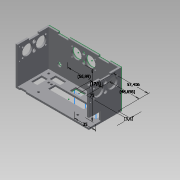
# Autodesk Inventor part: Kepala
Saved by Autodesk Inventor 2015 SP1 (Build 190203100, 203)
## iProperties
Created: 2015-02-01
Part Number: Kepala
Material: Generic
Document SubType Name: Modeling
Designer: Rafi Kurnia Putra
Density: 1 g/cm^3
Appearance: Default
Mass: 66.641 g
Surface Area: 406.742 cm^2
Volume: 66.641 cm^3
Author: Rafi Kurnia Putra
Autodesk Inventor part; units mm, degrees
ref_plane "YZ Plane" through (0, 0, 0) normal (1, 0, 0) x (0, 1, 0)
ref_plane "XY Plane" through (0, 0, 0) normal (0, 0, 1) x (1, 0, 0)
sketch "Sketch1" plane through (0, 0, 0) normal (0, 1, 0) x (-1, 0, 0)
  line L0 (60.406, -27.1071) -> (-60.406, -27.1071)
  line L1 (-60.406, -27.1071) -> (-60.406, 27.1071)
  line L2 (-60.406, 27.1071) -> (60.406, 27.1071)
  line L3 (60.406, 27.1071) -> (60.406, -27.1071)
  line L4 (60.406, -27.1071) -> (-60.406, 27.1071) construction
  line L5 (-60.406, -27.1071) -> (60.406, 27.1071) construction
  line L6 (-57.406, 24.1071) -> (-57.406, -27.1071)
  line L7 (57.406, -27.1071) -> (57.406, 24.1071)
  line L8 (57.406, 24.1071) -> (-57.406, 24.1071)
  point P0 (0, 0)
  point P1 (0, 0)
  dimension "d49" = 120.812
  dimension "d51" = 3
  dimension "d57" = 3
  dimension "d58" = 3
  dimension "d59" = 114.812
  dimension "d61" = 51.2141
  constraints: 18 end point, 3 midpoint, 3 parallel, 2 point on line, 1 horizontal, 1 perpendicular, 1 other
  measures "d49" distance of L1.end L2.end
  measures "d51" distance between parallel lines of L6 L1
  measures "d57" distance between parallel lines of L7 L3
  measures "d58" distance between parallel lines of L8 L2
  measures "d59" distance between parallel lines of L7 L6
  measures "d61" distance between parallel lines of L8 L0
extrude "Extrusion5" add sketch "Sketch1" against normal blind 3
extrude "Extrusion6" add sketch "Sketch1" along normal blind 60 contours L0 L7 L8 L6 L1 L2 L3
sketch "Sketch6" plane through (0, -3, 0) normal (0, -1, 0) x (1, 0, 0)
  circle A0 centre (-50.5965, 17.5471) radius 1.75
  circle A1 centre (50.5965, 17.5471) radius 1
  circle A2 centre (50.5965, 17.5471) radius 1.75
  circle A3 centre (-50.5965, 17.5471) radius 1.75
  point P0 (0, 0)
  dimension "d62" = 3.5
  constraints: 4 centre point, 2 coincident, 1 concentric, 4 other
  measures "d62" diameter of A2
extrude "Extrusion7" cut sketch "Sketch6" against normal up to next contours A0 | A1 | A2
sketch "Sketch7" plane through (0, -3, 0) normal (0, -1, 0) x (1, 0, 0)
  line L0 (-53.556, -8.4641) -> (-43.556, -8.4641)
  line L1 (-43.556, -8.4641) -> (-43.556, 9.0359)
  line L2 (-43.556, 9.0359) -> (-53.556, 9.0359)
  line L3 (-53.556, 9.0359) -> (-53.556, -8.4641)
  line L4 (-53.556, -8.4641) -> (-43.556, 9.0359) construction
  line L5 (-43.556, -8.4641) -> (-53.556, 9.0359) construction
  line L6 (53.556, -8.4641) -> (43.556, -8.4641)
  line L7 (43.556, -8.4641) -> (43.556, 9.0359)
  line L8 (43.556, 9.0359) -> (53.556, 9.0359)
  line L9 (53.556, 9.0359) -> (53.556, -8.4641)
  line L10 (53.556, -8.4641) -> (43.556, 9.0359) construction
  line L11 (43.556, -8.4641) -> (53.556, 9.0359) construction
  line L12 (-42.0848, 10.5071) -> (-24.5848, 10.5071)
  line L13 (-24.5848, 10.5071) -> (-24.5848, 20.5071)
  line L14 (-24.5848, 20.5071) -> (-42.0848, 20.5071)
  line L15 (-42.0848, 20.5071) -> (-42.0848, 10.5071)
  line L16 (-42.0848, 10.5071) -> (-24.5848, 20.5071) construction
  line L17 (-24.5848, 10.5071) -> (-42.0848, 20.5071) construction
  line L18 (42.0848, 10.5071) -> (24.5848, 10.5071)
  line L19 (24.5848, 10.5071) -> (24.5848, 20.5071)
  line L20 (24.5848, 20.5071) -> (42.0848, 20.5071)
  line L21 (42.0848, 20.5071) -> (42.0848, 10.5071)
  line L22 (42.0848, 10.5071) -> (24.5848, 20.5071) construction
  line L23 (24.5848, 10.5071) -> (42.0848, 20.5071) construction
  point P0 (0, 0)
  point P1 (-48.556, 0.2859)
  point P2 (-48.556, 0.2859)
  point P3 (48.556, 0.2859)
  point P4 (48.556, 0.2859)
  point P5 (-33.3348, 15.5071)
  point P6 (-33.3348, 15.5071)
  point P7 (33.3348, 15.5071)
  point P8 (33.3348, 15.5071)
  dimension "d65" = 10
  dimension "d66" = 17.5
  dimension "d69" = 10
  constraints: 48 end point, 10 midpoint, 4 parallel, 2 horizontal, 2 perpendicular
  measures "d65" distance of L2.end L1.end
  measures "d66" distance of L1.end L0.end
  measures "d69" distance of L13.end L12.end
extrude "Extrusion8" cut sketch "Sketch7" against normal up to next
sketch "Sketch9" plane through (0, 60, 0) normal (0, 1, 0) x (1, 0, 0)
  line L0 (60.406, 8.4641) -> (56.906, 8.4641)
  line L1 (56.906, -9.0359) -> (60.406, -9.0359)
  line L2 (60.406, 8.4641) -> (60.406, -9.0359)
  line L3 (56.906, -9.0359) -> (56.906, 8.4641)
  line L4 (42.0848, -23.8571) -> (42.0848, -27.3571)
  line L5 (42.0848, -27.3571) -> (24.5848, -27.3571)
  line L6 (24.5848, -23.8571) -> (42.0848, -23.8571)
  line L7 (24.5848, -23.8571) -> (24.5848, -27.3571)
  line L8 (0, 0) -> (0, -13)
  line L9 (-60.406, 8.4641) -> (-56.906, 8.4641)
  line L10 (-56.906, -9.0359) -> (-60.406, -9.0359)
  line L11 (-60.406, 8.4641) -> (-60.406, -9.0359)
  line L12 (-56.906, -9.0359) -> (-56.906, 8.4641)
  line L13 (-42.0848, -23.8571) -> (-42.0848, -27.3571)
  line L14 (-42.0848, -27.3571) -> (-24.5848, -27.3571)
  line L15 (-24.5848, -23.8571) -> (-42.0848, -23.8571)
  line L16 (-24.5848, -23.8571) -> (-24.5848, -27.3571)
  constraints: 34 end point, 8 symmetric about line, 2 vertical, 1 horizontal, 1 parallel
extrude "Extrusion9" cut sketch "Sketch9" against normal blind 3
sketch "Sketch10" plane through (0, -3, 0) normal (0, -1, 0) x (1, 0, 0)
  circle A0 centre (-32.4485, -17.4559) radius 1.75
  circle A1 centre (-37.593, 4.5441) radius 1.75
  circle A2 centre (32.4355, -17.4559) radius 1.75
  circle A3 centre (37.593, 4.5441) radius 1.75
  point P0 (0, 0)
  dimension "d84" = 22
  dimension "d85" = 22
  constraints: 4 centre point, 4 other
  measures "d84" vertical distance of A1.centre A0.centre
  measures "d85" vertical distance of A3.centre A2.centre
extrude "Extrusion10" cut sketch "Sketch10" against normal up to next
sketch "Sketch12" plane through (-60.406, -3, -27.1071) normal (-1, 0, 0) x (0, 0, 1)
  circle A0 centre (3, 59.0338) radius 1
  circle A1 centre (3, 38.0338) radius 1
  arc A2 (6.0857, 8.75) -> (6.7857, 8.05) centre (6.7857, 8.75) ccw
  arc A3 (13.0857, 8.05) -> (13.7857, 8.75) centre (13.0857, 8.75) ccw
  line L0 (13.0857, 8.05) -> (6.7857, 8.05)
  arc A4 (7.3007, 11.65) -> (6.9007, 11.25) centre (7.3007, 11.25) ccw
  arc A5 (12.9707, 11.25) -> (12.5707, 11.65) centre (12.5707, 11.25) ccw
  line L1 (7.3007, 11.25) -> (13.0857, 8.75) construction
  line L2 (13.0857, 8.75) -> (6.7857, 8.75) construction
  line L3 (6.7857, 8.75) -> (12.5707, 11.25) construction
  line L4 (2.4357, 5.1113) -> (17.4357, 5.1113)
  line L5 (17.4357, 5.1113) -> (17.4357, 15.1113)
  line L6 (17.4357, 15.1113) -> (2.4357, 15.1113)
  line L7 (2.4357, 15.1113) -> (2.4357, 5.1113)
  line L8 (2.4357, 5.1113) -> (17.4357, 15.1113) construction
  line L9 (17.4357, 5.1113) -> (2.4357, 15.1113) construction
  point P0 (27.1071, 3)
  point P1 (9.9357, 10.1113)
  dimension "d86" = 15
  dimension "d87" = 10
  constraints: 20 end point, 8 point on circle, 6 centre point, 3 horizontal, 2 midpoint, 2 parallel, 2 point on line, 1 perpendicular, 20 other
  measures "d86" distance of L6.end L5.end
  measures "d87" distance of L5.end L4.end
extrude "Extrusion11" cut sketch "Sketch12" against normal blind 200 contours A0 | A1
extrude "Extrusion12" cut sketch "Sketch12" against normal up to next contours L7 L6 L5 L4
fillet "Fillet2" radius 2 4 edges at (-58.906, 12.1113, -24.6713) (-58.906, 12.1113, -9.6713) (-58.906, 2.1113, -24.6713) (-58.906, 2.1113, -9.6713)
sketch "Sketch13" plane through (0, -3, 0) normal (0, -1, 0) x (1, 0, 0)
  line L0 (29.3575, 1.3171) -> (-29.3575, 1.3171)
  circle A0 centre (-32.8575, 4.3056) radius 1.75
  circle A1 centre (32.8575, 4.3056) radius 1.75
  line L1 (29.3575, 1.3171) -> (29.3575, 7.2941)
  line L2 (-29.3575, 1.3171) -> (-29.3575, 7.2941)
  line L3 (-29.3575, 7.2941) -> (29.3575, 7.2941)
  line L4 (-16, -57.1829) -> (-36, -57.1829)
  line L5 (-36, -57.1829) -> (-36, -2.1829)
  line L6 (-36, -2.1829) -> (-16, -2.1829)
  line L7 (-16, -2.1829) -> (-16, -57.1829)
  line L8 (-16, -57.1829) -> (-36, -2.1829) construction
  line L9 (-36, -57.1829) -> (-16, -2.1829) construction
  point P0 (0, 0)
  point P1 (34.6075, 4.3056)
  point P2 (29.3575, 4.3056)
  point P3 (-26, -29.6829)
  dimension "d96" = 3.5
  dimension "d95" = 3.5
  dimension "d97" = 3.5
  dimension "d99" = 20
  dimension "d100" = 55
  dimension "d101" = 3.5
  constraints: 20 end point, 3 horizontal, 3 perpendicular, 2 midpoint, 2 parallel, 1 centre point, 1 horizontal alignment, 3 other
  measures "d95" diameter of A0
  measures "d97" distance of point (32.857, 4.306) point (29.357, 4.306)
  measures "d99" distance of L5.end L6.end
  measures "d100" distance of L4.end L5.end
  measures "d101" distance between parallel lines of L0 L6
extrude "Extrusion13" cut sketch "Sketch13" against normal up to next contours L0 L2 L3 L1 | A0 | A1
ref_plane "Work Plane1" through (0, 19.75, 0) normal (0, 1, 0) x (-1, 0, 0)
sketch "Sketch20" plane through (-60.406, -3, -27.1071) normal (-1, 0, 0) x (0, 0, 1)
  line L0 (30.5999, 17.25) -> (30.5999, 19.25) projected
  arc A0 (31.0999, 19.75) -> (30.5999, 19.25) centre (31.0999, 19.25) ccw projected
  line L1 (31.0999, 19.75) -> (32.0999, 19.75) projected
  arc A1 (32.5999, 19.25) -> (32.0999, 19.75) centre (32.0999, 19.25) ccw projected
  line L2 (32.5999, 19.25) -> (32.5999, 17.25) projected
  line L3 (32.0999, 16.75) -> (31.0999, 16.75) projected
  arc A2 (30.5999, 17.25) -> (31.0999, 16.75) centre (31.0999, 17.25) ccw projected
  circle A3 centre (25.0999, 18.25) radius 3.75 projected
  arc A4 (32.0999, 16.75) -> (32.5999, 17.25) centre (32.0999, 17.25) ccw projected
  line L4 (31.0999, 19.25) -> (32.0999, 17.25) construction
  line L5 (32.0999, 17.25) -> (32.0999, 19.25) construction
  line L6 (30.5999, 19.25) -> (30.5999, 17.25) construction
  line L7 (32.0999, 19.25) -> (31.0999, 17.25) construction
  point P0 (27.1071, 3)
  point P1 (31.5999, 18.25)
  dimension "d132" = 6.5
  constraints: 6 end point, 1 midpoint, 1 parallel
  measures "d132" distance of point (31.6, 18.25) A3.centre
sketch "Sketch22" plane through (60.406, -3, 27.1071) normal (1, 0, 0) x (0, 0, -1)
  circle A0 centre (15.1412, 47.6838) radius 8.5
  circle A1 centre (38.0012, 47.6838) radius 8.5
  circle A2 centre (26.5712, 41.1438) radius 3
  circle A3 centre (45.6552, 40.0298) radius 1.6
  circle A4 centre (45.6552, 55.3378) radius 1.6
  circle A5 centre (7.4872, 55.3378) radius 1.6
  circle A6 centre (7.4872, 40.0298) radius 1.6
  circle A7 centre (26.5712, 54.2238) radius 3 projected
  point P0 (27.1071, 3)
  constraints: 7 centre point, 14 other
extrude "Extrusion24" cut sketch "Sketch22" against normal through all
sketch "Sketch23" plane through (-60.406, -3, 27.1071) normal (0, 0, 1) x (1, 0, 0)
  circle A0 centre (48.976, 47.6838) radius 8.5
  circle A1 centre (71.836, 47.6838) radius 8.5
  circle A2 centre (60.406, 41.1438) radius 3
  circle A3 centre (60.406, 54.2238) radius 3 projected
  circle A4 centre (79.49, 55.3378) radius 1.6
  circle A5 centre (79.49, 40.0298) radius 1.6
  circle A6 centre (41.322, 40.0298) radius 1.6
  circle A7 centre (41.322, 55.3378) radius 1.6
  point P0 (60.406, 3)
  constraints: 7 centre point, 14 other
extrude "Extrusion25" cut sketch "Sketch23" against normal up to next
sketch "Sketch24" plane through (0, -3, 0) normal (0, -1, 0) x (1, 0, 0)
  line L0 (53.556, -27.1071) -> (53.556, -43.2141)
  line L1 (43.556, -43.2141) -> (43.556, -27.1071)
  line L2 (53.556, -43.2141) -> (43.556, -43.2141)
  line L3 (53.556, -43.2141) -> (53.556, -25.7141)
  line L4 (53.556, -25.7141) -> (43.556, -25.7141)
  line L5 (43.556, -25.7141) -> (43.556, -27.1071)
  point P0 (0, 0)
  dimension "d164" = 17.5
  constraints: 12 end point, 3 vertical, 2 perpendicular, 1 horizontal, 4 other
  measures "d164" distance of L0.end L3.end
extrude "Extrusion26" cut sketch "Sketch24" against normal up to next
sketch "Sketch25" plane through (-60.406, -3, 27.1071) normal (0, 0, 1) x (1, 0, 0)
  line L0 (120.812, 22) -> (120.812, 14.5) projected
  line L1 (0, 63) -> (0, 0) projected
  line L2 (120.812, 18.25) -> (241.624, 18.25) construction
  circle A0 centre (41.322, 40.0298) radius 1.6 projected
  line L3 (41.322, 40.0298) -> (41.322, 18.25)
  circle A1 centre (79.49, 40.0298) radius 1.6 projected
  line L4 (79.49, 40.0298) -> (79.49, 18.25)
  line L5 (120.812, 18.25) -> (79.49, 18.25)
  line L6 (41.322, 18.25) -> (0, 18.25)
  circle A2 centre (100.151, 18.25) radius 3.75
  circle A3 centre (20.661, 18.25) radius 3.75
  point P0 (60.406, 3)
  dimension "d168" = 7.5
  dimension "d169" = 7.5
  constraints: 10 end point, 4 perpendicular, 3 midpoint, 2 centre point, 1 horizontal, 1 point on line
  measures "d168" diameter of A2
  measures "d169" diameter of A3
extrude "Extrusion27" cut sketch "Sketch25" against normal up to next contours A3 L6 | L6 A3 | A2 L5 | L5 A2
sketch "Sketch26" plane through (-60.406, -3, 27.1071) normal (0, 0, 1) x (1, 0, 0)
  circle A0 centre (20.661, 18.25) radius 3.75 projected
  circle A1 centre (100.151, 18.25) radius 3.75 projected
  line L0 (9.411, 28.5) -> (31.911, 28.5)
  line L1 (31.911, 28.5) -> (31.911, 25.5)
  line L2 (31.911, 25.5) -> (9.411, 25.5)
  line L3 (9.411, 25.5) -> (9.411, 28.5)
  line L4 (9.411, 28.5) -> (31.911, 25.5) construction
  line L5 (31.911, 28.5) -> (9.411, 25.5) construction
  line L6 (88.901, 28.5) -> (111.401, 28.5)
  line L7 (111.401, 28.5) -> (111.401, 25.5)
  line L8 (111.401, 25.5) -> (88.901, 25.5)
  line L9 (88.901, 25.5) -> (88.901, 28.5)
  line L10 (88.901, 28.5) -> (111.401, 25.5) construction
  line L11 (111.401, 28.5) -> (88.901, 25.5) construction
  point P0 (60.406, 3)
  point P1 (20.661, 27)
  point P2 (100.151, 27)
  dimension "d172" = 22.5
  dimension "d173" = 3
  dimension "d174" = 22.5
  constraints: 24 end point, 4 midpoint, 4 parallel, 2 horizontal, 2 perpendicular
  measures "d172" distance of L1.end L2.end
  measures "d173" distance of L0.end L1.end
  measures "d174" distance of L7.end L8.end
extrude "Extrusion28" add sketch "Sketch26" along normal blind 15 contours L0 L1 L2 L3 | L6 L7 L8 L9
sketch "Sketch27" plane through (-50.995, 25.5, 27.1071) normal (0, 1, 0) x (1, 0, 0)
  circle A0 centre (-13.5951, 23.8524) radius 3.75 projected
  line L0 (0, 0) -> (22.5, 0) projected
  line L1 (0, 0) -> (0, -15) projected
  line L2 (22.5, -15) -> (0, -15) projected
  line L3 (22.5, 0) -> (22.5, -15) projected
  line L4 (79.49, 0) -> (101.99, 0) projected
  line L5 (79.49, 0) -> (79.49, -15) projected
  line L6 (101.99, -15) -> (79.49, -15) projected
  line L7 (101.99, 0) -> (101.99, -15) projected
  circle A1 centre (11.25, -7.5) radius 3.75
  circle A2 centre (90.74, -7.5) radius 3.75
  point P0 (50.995, 27.1071)
  dimension "d177" = 7.5
  dimension "d178" = 7.5
  constraints: 2 centre point
  measures "d177" diameter of A1
  measures "d178" diameter of A2
extrude "Extrusion29" cut sketch "Sketch27" against normal up to next contours A1 | A2
sketch "Sketch30" plane through (28.495, 25.5, 27.1071) normal (0, 1, 0) x (1, 0, 0)
  circle A0 centre (-68.24, -7.5) radius 3.75 projected
  circle A1 centre (11.25, -7.5) radius 3.75 projected
  line L0 (17.25, -9) -> (18.25, -9)
  line L1 (18.75, -8.5) -> (18.75, -6.5)
  line L2 (18.25, -6) -> (17.25, -6)
  line L3 (16.75, -6.5) -> (16.75, -8.5)
  line L4 (16.75, -9) -> (18.75, -6) construction
  line L5 (18.75, -9) -> (16.75, -6) construction
  line L6 (4.25, -9) -> (5.25, -9)
  line L7 (5.75, -8.5) -> (5.75, -6.5)
  line L8 (5.25, -6) -> (4.25, -6)
  line L9 (3.75, -6.5) -> (3.75, -8.5)
  line L10 (3.75, -9) -> (5.75, -6) construction
  line L11 (5.75, -9) -> (3.75, -6) construction
  line L12 (-62.24, -9) -> (-61.24, -9)
  line L13 (-60.74, -8.5) -> (-60.74, -6.5)
  line L14 (-61.24, -6) -> (-62.24, -6)
  line L15 (-62.74, -6.5) -> (-62.74, -8.5)
  line L16 (-62.74, -9) -> (-60.74, -6) construction
  line L17 (-60.74, -9) -> (-62.74, -6) construction
  line L18 (-74.24, -9) -> (-75.24, -9)
  line L19 (-75.74, -8.5) -> (-75.74, -6.5)
  line L20 (-75.24, -6) -> (-74.24, -6)
  line L21 (-73.74, -6.5) -> (-73.74, -8.5)
  line L22 (-73.74, -9) -> (-75.74, -6) construction
  line L23 (-75.74, -9) -> (-73.74, -6) construction
  arc A2 (-75.24, -6) -> (-75.74, -6.5) centre (-75.24, -6.5) ccw
  arc A3 (-73.74, -6.5) -> (-74.24, -6) centre (-74.24, -6.5) ccw
  arc A4 (-74.24, -9) -> (-73.74, -8.5) centre (-74.24, -8.5) ccw
  arc A5 (-75.74, -8.5) -> (-75.24, -9) centre (-75.24, -8.5) ccw
  arc A6 (-61.24, -9) -> (-60.74, -8.5) centre (-61.24, -8.5) ccw
  arc A7 (-60.74, -6.5) -> (-61.24, -6) centre (-61.24, -6.5) ccw
  arc A8 (-62.24, -6) -> (-62.74, -6.5) centre (-62.24, -6.5) ccw
  arc A9 (-62.74, -8.5) -> (-62.24, -9) centre (-62.24, -8.5) ccw
  arc A10 (16.75, -8.5) -> (17.25, -9) centre (17.25, -8.5) ccw
  arc A11 (17.25, -6) -> (16.75, -6.5) centre (17.25, -6.5) ccw
  arc A12 (18.75, -6.5) -> (18.25, -6) centre (18.25, -6.5) ccw
  arc A13 (18.25, -9) -> (18.75, -8.5) centre (18.25, -8.5) ccw
  arc A14 (5.25, -9) -> (5.75, -8.5) centre (5.25, -8.5) ccw
  arc A15 (5.75, -6.5) -> (5.25, -6) centre (5.25, -6.5) ccw
  arc A16 (4.25, -6) -> (3.75, -6.5) centre (4.25, -6.5) ccw
  arc A17 (3.75, -8.5) -> (4.25, -9) centre (4.25, -8.5) ccw
  point P0 (-28.495, 27.1071)
  point P1 (17.75, -7.5)
  point P2 (4.75, -7.5)
  point P3 (-61.74, -7.5)
  point P4 (-74.74, -7.5)
  dimension "d187" = 2
  dimension "d188" = 3
  dimension "d189" = 6.5
  dimension "d190" = 2
  dimension "d191" = 3
  dimension "d192" = 6.5
  dimension "d193" = 2
  dimension "d194" = 3
  dimension "d195" = 2
  dimension "d196" = 3
  dimension "d197" = 6.5
  dimension "d198" = 6.5
  dimension "d199" = 0.5
  constraints: 48 end point, 32 point on circle, 32 point on line, 32 tangent, 16 centre point, 15 equal radius, 8 midpoint, 8 parallel, 4 horizontal, 4 perpendicular
  measures "d187" distance of L5.end L4.end
  measures "d188" distance of L4.end L5.start
  measures "d189" distance of point (17.75, -7.5) A1.centre
  measures "d190" distance of L11.end L10.end
  measures "d191" distance of L10.end L11.start
  measures "d192" distance of point (4.75, -7.5) A1.centre
  measures "d193" distance of L17.end L16.end
  measures "d194" distance of L16.end L17.start
  measures "d195" distance of L22.end L23.end
  measures "d196" distance of L23.start L22.end
  measures "d197" distance of point (-74.74, -7.5) A0.centre
  measures "d198" distance of A0.centre point (-61.74, -7.5)
  measures "d199" radius of A2
extrude "Extrusion30" cut sketch "Sketch30" against normal up to next contours A10 L3 A11 L2 A12 L1 A13 L0 | A17 L9 A16 L8 A15 L7 A14 L6 | A9 L15 A8 L14 A7 L13 A6 L12 | L18 A5 L19 A2 L20 A3 L21 A4
chamfer "Chamfer1" distance 5 angle 45 4 edges at (-50.995, 24, 42.1071) (-28.495, 24, 42.1071) (28.495, 24, 42.1071) (50.995, 24, 42.1071)
sketch "Sketch34" plane through (-60.406, -3, -27.1071) normal (-1, 0, 0) x (0, 0, 1)
  circle A0 centre (39.0729, 47.6838) radius 8.5 projected
  circle A1 centre (27.6429, 41.1438) radius 3 projected
  circle A2 centre (46.7269, 55.3378) radius 1.6 projected
  circle A3 centre (8.5589, 40.0298) radius 1.6 projected
  circle A4 centre (8.5589, 55.3378) radius 1.6 projected
  circle A5 centre (46.7269, 40.0298) radius 1.6 projected
  circle A6 centre (27.6429, 54.2238) radius 3 projected
  circle A7 centre (16.2129, 47.6838) radius 8.5 projected
  line L0 (17.4357, 13.1113) -> (17.4357, 7.1113) projected
  arc A8 (15.4357, 5.1113) -> (17.4357, 7.1113) centre (15.4357, 7.1113) ccw projected
  line L1 (15.4357, 5.1113) -> (4.4357, 5.1113) projected
  arc A9 (2.4357, 7.1113) -> (4.4357, 5.1113) centre (4.4357, 7.1113) ccw projected
  line L2 (2.4357, 7.1113) -> (2.4357, 13.1113) projected
  arc A10 (4.4357, 15.1113) -> (2.4357, 13.1113) centre (4.4357, 13.1113) ccw projected
  line L3 (4.4357, 15.1113) -> (15.4357, 15.1113) projected
  arc A11 (17.4357, 13.1113) -> (15.4357, 15.1113) centre (15.4357, 13.1113) ccw projected
  circle A12 centre (3, 59.0338) radius 1 projected
  circle A13 centre (3, 38.0338) radius 1 projected
  line L4 (36.1429, 63) -> (36.1429, 60) projected
  line L5 (36.1429, 60) -> (18.6429, 60) projected
  line L6 (18.6429, 60) -> (18.6429, 63) projected
  line L7 (0, 63) -> (18.6429, 63) projected
  line L8 (0, 63) -> (0, 0) projected
  line L9 (54.2141, 0) -> (0, 0) projected
  line L10 (54.2141, 0) -> (54.2141, 63) projected
  line L11 (36.1429, 63) -> (54.2141, 63) projected
  line L12 (4.4357, 15.1113) -> (15.4357, 15.1113) projected
  arc A14 (4.4357, 15.1113) -> (2.4357, 13.1113) centre (4.4357, 13.1113) ccw projected
  line L13 (2.4357, 7.1113) -> (2.4357, 13.1113) projected
  arc A15 (2.4357, 7.1113) -> (4.4357, 5.1113) centre (4.4357, 7.1113) ccw projected
  line L14 (15.4357, 5.1113) -> (4.4357, 5.1113) projected
  arc A16 (15.4357, 5.1113) -> (17.4357, 7.1113) centre (15.4357, 7.1113) ccw projected
  line L15 (17.4357, 13.1113) -> (17.4357, 7.1113) projected
  arc A17 (17.4357, 13.1113) -> (15.4357, 15.1113) centre (15.4357, 13.1113) ccw projected
  line L16 (0, 3) -> (51.2141, 3) projected
  line L17 (19.8715, 17.2226) -> (0, 17.2226)
  line L18 (0, 17.2226) -> (0, 3)
  line L19 (0, 3) -> (19.8715, 3)
  line L20 (19.8715, 3) -> (19.8715, 17.2226)
  line L21 (19.8715, 17.2226) -> (0, 3) construction
  line L22 (0, 17.2226) -> (19.8715, 3) construction
  point P0 (27.1071, 3)
  point P1 (9.9357, 10.1113)
  constraints: 12 end point, 2 midpoint, 2 parallel, 1 horizontal, 1 perpendicular
extrude "Extrusion31" cut sketch "Sketch34" against normal blind 10 contours L0 A8 L1 A9 L2 A10 L3 A11 | L8 L17 L20 L16
sketch "Sketch35" plane through (0, 0, 0) normal (0, 1, 0) x (1, 0, 0)
  line L0 (-24.5848, -10.5071) -> (-24.5848, -20.5071) projected
  line L1 (-24.5848, -20.5071) -> (-42.0848, -20.5071) projected
  line L2 (-42.0848, -10.5071) -> (-24.5848, -10.5071) projected
  line L3 (-42.0848, -20.5071) -> (-42.0848, -10.5071) projected
  line L4 (-8.75, -10.5071) -> (8.75, -10.5071)
  line L5 (8.75, -10.5071) -> (8.75, -20.5071)
  line L6 (8.75, -20.5071) -> (-8.75, -20.5071)
  line L7 (-8.75, -20.5071) -> (-8.75, -10.5071)
  line L8 (-8.75, -10.5071) -> (8.75, -20.5071) construction
  line L9 (8.75, -10.5071) -> (-8.75, -20.5071) construction
  line L10 (29.3575, -1.3171) -> (29.3575, -7.2941) projected
  line L11 (-29.3575, -7.2941) -> (-29.3575, -1.3171) projected
  line L12 (29.3575, -1.3171) -> (-29.3575, -1.3171)
  line L13 (-29.3575, -1.3171) -> (-29.3575, 4.6829)
  line L14 (-29.3575, 4.6829) -> (29.3575, 4.6829)
  line L15 (29.3575, 4.6829) -> (29.3575, -1.3171)
  point P0 (0, 0)
  point P1 (0, -15.5071)
  dimension "d225" = 17.5
  dimension "d226" = 10
  dimension "d227" = 17.5
  dimension "d228" = 6
  constraints: 20 end point, 4 parallel, 2 horizontal, 2 midpoint, 2 perpendicular
  measures "d225" distance of L2.start L0.start
  measures "d226" distance between parallel lines of L2 L1
  measures "d227" distance of L5.end L6.end
  measures "d228" distance of L12.end L13.end
extrude "Extrusion32" cut sketch "Sketch35" against normal through all contours L4 L5 L6 L7 | L12 L13 L14 L15
sketch "Sketch36" plane through (0, -3, 0) normal (0, -1, 0) x (1, 0, 0)
  line L0 (-57.406, 24.1071) -> (57.406, 24.1071) projected
  line L1 (-57.406, -7.2356) -> (-57.406, 24.1071) projected
  line L2 (-8.75, 20.5071) -> (8.75, 20.5071) projected
  line L3 (8.75, 10.5071) -> (-8.75, 10.5071) projected
  line L4 (-8.75, 10.5071) -> (-8.75, 20.5071) projected
  line L5 (8.75, 20.5071) -> (8.75, 10.5071) projected
  point P0 (0, 0)
  point P1 (0, 15.5071)
  dimension "d231" = 3.6
  dimension "d232" = 48.656
  dimension "d233" = 17.5
  dimension "d234" = 57.406
  measures "d231" distance between parallel lines of L0 L2
  measures "d232" horizontal distance of L0.start L2.start
  measures "d233" distance of L2.start L2.end
  measures "d234" horizontal distance of L0.start point (0, 15.507)
sketch "Sketch37" plane through (-60.406, -3, 27.1071) normal (0, 0, 1) x (1, 0, 0)
  line L0 (31.911, 28.5) -> (31.911, 25.5) projected
  line L1 (31.911, 25.5) -> (9.411, 25.5) projected
  line L2 (9.411, 25.5) -> (9.411, 28.5) projected
  line L3 (9.411, 28.5) -> (31.911, 28.5) projected
  line L4 (111.401, 28.5) -> (111.401, 25.5) projected
  line L5 (111.401, 25.5) -> (88.901, 25.5) projected
  line L6 (88.901, 25.5) -> (88.901, 28.5) projected
  line L7 (88.901, 28.5) -> (111.401, 28.5) projected
  circle A0 centre (100.151, 18.25) radius 3.75 projected
  circle A1 centre (20.661, 18.25) radius 3.75 projected
  circle A2 centre (48.976, 47.6838) radius 8.5 projected
  circle A3 centre (60.406, 41.1438) radius 3 projected
  circle A4 centre (41.322, 40.0298) radius 1.6 projected
  circle A5 centre (79.49, 55.3378) radius 1.6 projected
  circle A6 centre (79.49, 40.0298) radius 1.6 projected
  circle A7 centre (41.322, 55.3378) radius 1.6 projected
  circle A8 centre (60.406, 54.2238) radius 3 projected
  circle A9 centre (71.836, 47.6838) radius 8.5 projected
  line L8 (84.9908, 60) -> (84.9908, 63) projected
  line L9 (35.8212, 63) -> (84.9908, 63) projected
  line L10 (35.8212, 63) -> (35.8212, 60) projected
  line L11 (35.8212, 60) -> (18.3212, 60) projected
  line L12 (18.3212, 60) -> (18.3212, 63) projected
  line L13 (0, 63) -> (18.3212, 63) projected
  line L14 (0, 0) -> (0, 63) projected
  line L15 (120.812, 0) -> (0, 0) projected
  line L16 (120.812, 0) -> (120.812, 63) projected
  line L17 (102.4908, 63) -> (120.812, 63) projected
  line L18 (102.4908, 63) -> (102.4908, 60) projected
  line L19 (102.4908, 60) -> (84.9908, 60) projected
  line L20 (60.406, 35.5) -> (60.406, -39.5)
  line L21 (42.906, 35.5) -> (42.906, -39.5)
  line L22 (42.906, -39.5) -> (77.906, -39.5)
  line L23 (77.906, -39.5) -> (77.906, 35.5)
  line L24 (77.906, 35.5) -> (42.906, 35.5)
  point P0 (60.406, 3)
  dimension "d235" = 56.99
  dimension "d236" = 75
  dimension "d237" = 35
  constraints: 10 end point, 2 parallel, 2 vertical, 1 perpendicular
  measures "d235" distance between parallel lines of L6 L0
  measures "d236" distance of L20.start L20.end
  measures "d237" distance of L22.end L21.end
body "Solid2"
